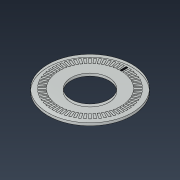
# Autodesk Inventor part: iC-Haus PX01S 26-360
Saved by Autodesk Inventor 2022.1 (Build 261234020, 234B)
## iProperties
Part Number: iC-Haus PX01S 26-360
Material: Glas
Document SubType Name: Modeling
Designer: rYan
Mass: 0.741786 g
Surface Area: 9.48238 cm^2
Volume: 0.340269 cm^3
Density: 2.18 g/cm^3
Appearance: Klar
Author: rYan
Autodesk Inventor part; units mm, degrees
ref_plane "YZ Plane" through (0, 0, 0) normal (1, 0, 0) x (0, 1, 0)
ref_plane "XZ Plane" through (0, 0, 0) normal (0, 1, 0) x (-1, 0, 0)
ref_plane "XY Plane" through (0, 0, 0) normal (0, 0, 1) x (1, 0, 0)
sketch "Skizze1" plane through (0, 0, 0) normal (0, 0, 1) x (1, 0, 0)
  circle A0 centre (0, 0) radius 5.85
  circle A1 centre (0, 0) radius 13
  dimension "d11" = 11.7
  dimension "d12" = 26
  constraints: 2 centre point, 2 coincident
  measures "d11" diameter of A0
  measures "d12" diameter of A1
extrude "Extrusion1" add sketch "Skizze1" against normal blind 0.8
sketch "Skizze2" plane through (0, 0, 0) normal (0, 0, 1) x (1, 0, 0)
  circle A0 centre (0, 0) radius 13 projected
  line L0 (-0.3, 11.5) -> (0.3, 11.5)
  line L1 (0.3, 11.5) -> (0.3, 9.5)
  line L2 (0.3, 9.5) -> (-0.3, 9.5)
  line L3 (-0.3, 9.5) -> (-0.3, 11.5)
  line L4 (0, 18.2) -> (0, -18.2) projected
  dimension "d4" = 2
  dimension "d5" = 0.6
  dimension "d13" = 1.5
  constraints: 8 end point, 2 parallel, 1 horizontal, 1 perpendicular, 1 other
  measures "d4" distance of L0.end L1.end
  measures "d5" distance of L1.end L2.end
  measures "d13" distance edge to line of A0 L0
extrude "Extrusion2" add sketch "Skizze2" along normal blind 0.02 contours L4 L2 L3 L0 | L0 L1 L2 L4
pattern_circular "Runde Anordnung1" count 64 over 360 about axis through (0, 0, -10) along (0, 0, 1) of "Extrusion2"
